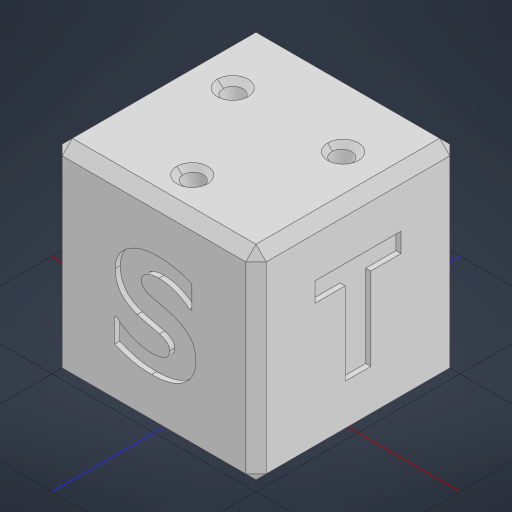
# Autodesk Inventor part: DartCube_Stef
Saved by Autodesk Inventor 2023.2 (Build 272271030, 271C)
## iProperties
Created: 2023-05-18
Part Number: DartCube_Stef
Material: Generisch
Document SubType Name: Modeling
Designer: Stefan
Mass: 61.7619 g
Surface Area: 101.076 cm^2
Volume: 61.7619 cm^3
Density: 1 g/cm^3
Appearance: Vorgabe
Author: Stefan
Autodesk Inventor part; units mm, degrees
ref_plane "YZ Plane" through (0, 0, 0) normal (1, 0, 0) x (0, 1, 0)
ref_plane "XZ Plane" through (0, 0, 0) normal (0, 1, 0) x (-1, 0, 0)
sketch "Skizze1" plane through (0, 0, 0) normal (0, 1, 0) x (-1, 0, 0)
  line L0 (-20, 20) -> (20, 20)
  line L1 (20, 20) -> (20, -20)
  line L2 (20, -20) -> (-20, -20)
  line L3 (-20, -20) -> (-20, 20)
  line L4 (-20, 20) -> (20, -20) construction
  line L5 (20, 20) -> (-20, -20) construction
  point P0 (0, 0)
  dimension "d0" = 40
  constraints: 12 end point, 2 midpoint, 2 parallel, 2 perpendicular, 1 horizontal
  measures "d0" distance of L1.end L2.end
extrude "Extrusion1" add sketch "Skizze1" along normal blind 40
ref_plane "Arbeitsebene2" through (0, 13, 0) normal (0, 1, 0) x (1, 0, 0)
sketch "Skizze8" plane through (0, 40, 0) normal (0, 1, 0) x (1, 0, 0)
  circle A0 centre (0, 0) radius 12.5 construction
  circle A1 centre (0, -12.5) radius 2
  circle A2 centre (10.8253, 6.25) radius 2
  circle A3 centre (-10.8253, 6.25) radius 2
  dimension "d32" = 25
  dimension "d33" = 4
  dimension "d36" = 360
  constraints: 3 centre point, 2 vertical alignment, 1 coincident, 9 other
  measures "d33" diameter of A1
sketch "Skizze9" plane through (0, 13, 0) normal (0, 1, 0) x (1, 0, 0)
  circle A0 centre (0, 0) radius 7.5 construction
  circle A1 centre (0, -7.5) radius 1
  circle A2 centre (6.4952, 3.75) radius 1
  circle A3 centre (-6.4952, 3.75) radius 1
  dimension "d38" = 15
  dimension "d39" = 2
  dimension "d42" = 360
  constraints: 3 centre point, 2 vertical alignment, 1 coincident, 9 other
  measures "d39" diameter of A1
loft "Erhebung1" cut profiles "Skizze8", "Skizze9" contours A1 / A1
loft "Erhebung2" cut profiles "Skizze8", "Skizze9" contours A2 / A2
loft "Erhebung3" cut profiles "Skizze8", "Skizze9" contours A3 / A3
chamfer "Fase1" distance 2 angle 45 12 edges at (20, 20, 20) (20, 40, 0) (0, 40, 20) (0, 40, -20) (20, 20, -20) (0, 0, -20) (20, 0, 0) (-20, 20, -20) (-20, 0, 0) (-20, 40, 0) (-20, 20, 20) (0, 0, 20)
chamfer "Fase2" distance 1 angle 45 3 edges at (-2, 40, 12.5) (-12.8253, 40, -6.25) (8.8253, 40, -6.25)
sketch "Skizze4" plane through (20, 2, 20) normal (0, 0, 1) x (1, 0, 0)
  line L0 (-38, 36) -> (-2, 36) construction
  line L1 (-2, 36) -> (-2, 0) construction
  line L2 (-2, 0) -> (-38, 0) construction
  line L3 (-38, 0) -> (-38, 36) construction
  line L4 (0, 0) -> (0, 0) projected
  line L5 (-38, 36) -> (-2, 36) projected
  line L6 (-2, 36) -> (-2, 0) projected
  line L7 (-2, 0) -> (-38, 0) projected
  line L8 (-38, 0) -> (-38, 36) projected
  spline S0 degree 2 poles (-20.4619, 7.6434) (-22.7634, 7.6434) (-26.2318, 8.5348) (-27.7229, 9.1831) knots 0 0 0 1 2 2 2
  line L9 (-27.7229, 9.1831) -> (-27.7229, 13.9481)
  line L10 (-27.7229, 13.9481) -> (-27.269, 13.9481)
  spline S1 degree 2 poles (-27.269, 13.9481) (-25.7618, 12.6677) (-22.1475, 11.2901) (-20.4457, 11.2901) knots 0 0 0 1 2 2 2
  spline S2 degree 2 poles (-20.4457, 11.2901) (-20.0081, 11.2901) (-18.5981, 11.4846) (-18.1767, 11.6791) knots 0 0 0 1 2 2 2
  spline S3 degree 2 poles (-18.1767, 11.6791) (-17.658, 11.906) (-16.9287, 12.7326) (-16.9287, 13.3971) knots 0 0 0 1 2 2 2
  spline S4 degree 2 poles (-16.9287, 13.3971) (-16.9287, 14.1588) (-18.1118, 15.0989) (-18.9222, 15.3096) knots 0 0 0 1 2 2 2
  spline S5 degree 2 poles (-18.9222, 15.3096) (-19.9433, 15.5851) (-22.2609, 16.0551) (-23.282, 16.4117) knots 0 0 0 1 2 2 2
  spline S6 degree 2 poles (-23.282, 16.4117) (-25.5997, 17.222) (-27.6094, 19.9935) (-27.6094, 22.0681) knots 0 0 0 1 2 2 2
  spline S7 degree 2 poles (-27.6094, 22.0681) (-27.6094, 24.872) (-22.8606, 28.3566) (-19.295, 28.3566) knots 0 0 0 1 2 2 2
  spline S8 degree 2 poles (-19.295, 28.3566) (-17.5122, 28.3566) (-13.9789, 27.6272) (-12.5851, 27.0113) knots 0 0 0 1 2 2 2
  line L11 (-12.5851, 27.0113) -> (-12.5851, 22.4408)
  line L12 (-12.5851, 22.4408) -> (-13.0227, 22.4408)
  spline S9 degree 2 poles (-13.0227, 22.4408) (-14.141, 23.3971) (-17.3501, 24.7099) (-19.0357, 24.7099) knots 0 0 0 1 2 2 2
  spline S10 degree 2 poles (-19.0357, 24.7099) (-19.7002, 24.7099) (-20.7374, 24.5154) (-21.3209, 24.2561) knots 0 0 0 1 2 2 2
  spline S11 degree 2 poles (-21.3209, 24.2561) (-21.7909, 24.0454) (-22.4716, 23.2026) (-22.4716, 22.684) knots 0 0 0 1 2 2 2
  spline S12 degree 2 poles (-22.4716, 22.684) (-22.4716, 21.906) (-21.3857, 21.0146) (-19.8298, 20.658) knots 0 0 0 1 2 2 2
  spline S13 degree 2 poles (-19.8298, 20.658) (-18.825, 20.4311) (-16.9611, 19.9935) (-15.8914, 19.6207) knots 0 0 0 1 2 2 2
  spline S14 degree 2 poles (-15.8914, 19.6207) (-13.8169, 18.859) (-11.7909, 16.3306) (-11.7909, 14.2561) knots 0 0 0 1 2 2 2
  spline S15 degree 2 poles (-11.7909, 14.2561) (-11.7909, 11.2739) (-16.4749, 7.6434) (-20.4619, 7.6434) knots 0 0 0 1 2 2 2
  point P0 (-20, -2)
  dimension "d0" = 40
  constraints: 4 collinear, 2 other
sketch "Skizze5" plane through (20, 2, -20) normal (1, 0, 0) x (0, 0, -1)
  line L0 (-38, 36) -> (-2, 36) construction
  line L1 (-2, 36) -> (-2, 0) construction
  line L2 (-2, 0) -> (-38, 0) construction
  line L3 (-38, 0) -> (-38, 36) construction
  line L4 (0, 0) -> (0, 0) projected
  line L5 (-38, 0) -> (-38, 36) projected
  line L6 (-2, 0) -> (-38, 0) projected
  line L7 (-2, 36) -> (-2, 0) projected
  line L8 (-38, 36) -> (-2, 36) projected
  line L9 (-22.5122, 8) -> (-22.5122, 24.1912)
  line L10 (-22.5122, 24.1912) -> (-28.4279, 24.1912)
  line L11 (-28.4279, 24.1912) -> (-28.4279, 28)
  line L12 (-28.4279, 28) -> (-11.5721, 28)
  line L13 (-11.5721, 28) -> (-11.5721, 24.1912)
  line L14 (-11.5721, 24.1912) -> (-17.4878, 24.1912)
  line L15 (-17.4878, 24.1912) -> (-17.4878, 8)
  line L16 (-17.4878, 8) -> (-22.5122, 8)
  point P0 (-20, -2)
  dimension "d0" = 40
  constraints: 4 collinear, 2 other
sketch "Skizze6" plane through (-20, 2, -20) normal (0, 0, -1) x (-1, 0, 0)
  line L0 (-38, 36) -> (-2, 36) construction
  line L1 (-2, 36) -> (-2, 0) construction
  line L2 (-2, 0) -> (-38, 0) construction
  line L3 (-38, 0) -> (-38, 36) construction
  line L4 (0, 0) -> (0, 0) projected
  line L5 (-38, 36) -> (-2, 36) projected
  line L6 (-38, 0) -> (-38, 36) projected
  line L7 (-2, 0) -> (-38, 0) projected
  line L8 (-2, 36) -> (-2, 0) projected
  line L9 (-26.3857, 8) -> (-26.3857, 28)
  line L10 (-26.3857, 28) -> (-12.8687, 28)
  line L11 (-12.8687, 28) -> (-12.8687, 24.1912)
  line L12 (-12.8687, 24.1912) -> (-21.3938, 24.1912)
  line L13 (-21.3938, 24.1912) -> (-21.3938, 20.6742)
  line L14 (-21.3938, 20.6742) -> (-13.5332, 20.6742)
  line L15 (-13.5332, 20.6742) -> (-13.5332, 16.8655)
  line L16 (-13.5332, 16.8655) -> (-21.3938, 16.8655)
  line L17 (-21.3938, 16.8655) -> (-21.3938, 11.8088)
  line L18 (-21.3938, 11.8088) -> (-12.8687, 11.8088)
  line L19 (-12.8687, 11.8088) -> (-12.8687, 8)
  line L20 (-12.8687, 8) -> (-26.3857, 8)
  point P0 (-20, -2)
  dimension "d0" = 40
  constraints: 4 collinear, 2 other
sketch "Skizze7" plane through (-20, 2, 20) normal (-1, 0, 0) x (0, 0, 1)
  line L0 (-38, 36) -> (-2, 36) construction
  line L1 (-2, 36) -> (-2, 0) construction
  line L2 (-2, 0) -> (-38, 0) construction
  line L3 (-38, 0) -> (-38, 36) construction
  line L4 (0, 0) -> (0, 0) projected
  line L5 (-38, 36) -> (-2, 36) projected
  line L6 (-38, 0) -> (-38, 36) projected
  line L7 (-2, 0) -> (-38, 0) projected
  line L8 (-2, 36) -> (-2, 0) projected
  line L9 (-12.5284, 24.1912) -> (-20.9238, 24.1912)
  line L10 (-20.9238, 24.1912) -> (-20.9238, 20.4149)
  line L11 (-20.9238, 20.4149) -> (-13.1929, 20.4149)
  line L12 (-13.1929, 20.4149) -> (-13.1929, 16.6062)
  line L13 (-13.1929, 16.6062) -> (-20.9238, 16.6062)
  line L14 (-20.9238, 16.6062) -> (-20.9238, 8)
  line L15 (-20.9238, 8) -> (-25.9157, 8)
  line L16 (-25.9157, 8) -> (-25.9157, 28)
  line L17 (-25.9157, 28) -> (-12.5284, 28)
  line L18 (-12.5284, 28) -> (-12.5284, 24.1912)
  point P0 (-20, -2)
  dimension "d0" = 40
  constraints: 4 collinear, 2 other
emboss "Prägen1" sketch "Skizze4" operation cut depth 1 direction (0, 0, -1) contours S0 L9 L10 S1 S2 S3 S4 S5 S6 S7 S8 L11 L12 S9 S10 S11 S12 S13 S14 S15
emboss "Prägen2" sketch "Skizze5" operation cut depth 1 direction (-1, 0, 0) contours L9 L10 L11 L12 L13 L14 L15 L16
emboss "Prägen3" sketch "Skizze6" operation cut depth 1 direction (0, 0, 1) contours L9 L10 L11 L12 L13 L14 L15 L16 L17 L18 L19 L20
emboss "Prägen4" sketch "Skizze7" operation cut depth 1 direction (1, 0, 0) contours L9 L10 L11 L12 L13 L14 L15 L16 L17 L18
equation "\"d2\" = d0"
